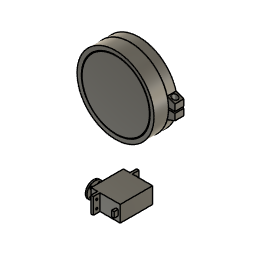
FlatPanel - SpaceCat51 v10 (Autodesk Fusion 360 design; units mm, degrees)
Autodesk Fusion 360 part; units mm, degrees
sketch "Sketch1" plane through (0, 0, 0) normal (0, 1, 0) x (1, 0, 0) in component "TelescopeBracket"
  circle A0 centre (0, 0) radius 40 construction
  circle A1 centre (0, 0) radius 42.4
  circle A2 centre (0, 0) radius 47.4
  line L0 (0, 0) -> (47.4, 0) construction
  line L1 (42.3882, -1) -> (48.4, -1)
  line L2 (48.4, -1) -> (48.4, 1)
  line L3 (48.4, 1) -> (42.3882, 1)
  line L4 (42.3882, 1) -> (42.3882, -1)
  line L5 (42.3882, -1) -> (55.3882, -1)
  line L6 (55.3882, -1) -> (55.3882, -4)
  line L7 (55.3882, -4) -> (42.3882, -4)
  line L8 (42.3882, -4) -> (42.3882, -1)
  line L9 (55.3882, -4) -> (42.3882, -4)
  line L10 (42.3882, -4) -> (42.3882, -9)
  line L11 (42.3882, -9) -> (55.3882, -9)
  line L12 (55.3882, -9) -> (55.3882, -4)
  line L13 (55.3882, -9) -> (45.7166, -12.5202)
  line L14 (55.3882, -9) -> (65.3491, -9) construction
  line L15 (42.3882, 1) -> (55.3882, 1)
  line L16 (55.3882, 1) -> (55.3882, 4)
  line L17 (55.3882, 9) -> (55.3882, 4)
  line L18 (55.3882, 9) -> (45.7166, 12.5202)
  dimension "d1" = 80
  dimension "d3" = 2.4
  dimension "d4" = 5
  dimension "d15" = 2
  dimension "d16" = 1
  dimension "d17" = 13
  dimension "d18" = 3
  dimension "d20" = 5
  dimension "d21" = 160
  constraint coincident A0.centre A1.centre
  constraint coincident A2 L0.end
  constraint horizontal L0
  constraint horizontal L1
  constraint vertical L2
  constraint horizontal L3
  constraint vertical L4
  constraint coincident A1 L1.start
  constraint horizontal L5
  constraint vertical L6
  constraint horizontal L7
  constraint vertical L8
  constraint horizontal L9
  constraint vertical L10
  constraint horizontal L11
  constraint vertical L12
  constraint horizontal L14
  constraint symmetric L0 L1.start L3.end
  constraint symmetric L0 L5.end L15.end
  constraint symmetric L0 L6.end L16.end
  constraint symmetric L0 L11.end L17.start
  constraint symmetric L0 L13.end L18.end
  constraint coincident A2 L13.end
  measures "d1" diameter of A0
  measures "d3" distance of A0 A1
  measures "d4" distance of A1 A2
  measures "d15" distance of L1 L3
  measures "d16" distance of L0 L1
  measures "d17" distance of L1.start L5.end
  measures "d18" distance of L5 L7
  measures "d20" distance of L6.end L11.end
  measures "d21" angle of L13 L14
extrude "Extrude2" add sketch "Sketch1" along normal blind 11 contours A1 A2 L3 L8 L10 L11 L15 | A2 L1 L5 L7 L8 L9 | A2 L3 L15 L16 L17 L18 | A2 L1 L5 L6 L7 L9 | A2 L7 L9 L10 L11 | A2 L7 L9 L11 L12 | A2 L11 L13 makes body 1 in component "TelescopeBracket"
sketch "Sketch2" plane through (0, 0, -1) normal (0, 0, 1) x (-1, 0, 0) in component "TelescopeBracket"
  line L0 (-42.3882, 0) -> (-55.3882, 0)
  line L1 (-55.3882, -11) -> (-42.3882, -11)
  line L2 (-42.3882, -11) -> (-42.3882, 0)
  circle A0 centre (-49.3882, -5.5) radius 3
  circle A1 centre (-49.3882, -5.5) radius 3
  line L3 (-55.3882, 0) -> (-55.3882, -11)
  dimension "d24" = 6
  dimension "d25" = 6
  dimension "d38" = 6
  dimension "d39" = 6
  dimension "d40" = 5.5
  dimension "d41" = 5.5
  measures "d24" diameter of A0
  measures "d25" diameter of A1
  measures "d38" distance of A0.centre L3
  measures "d39" distance of A0.centre L3
  measures "d40" distance of L0 A0.centre
  measures "d41" distance of L1 A0.centre
extrude "Extrude3" cut sketch "Sketch2" against normal blind 20 contours A0 A1 bodies 1 in component "TelescopeBracket"
sketch "Sketch3" plane through (0, 0, 1) normal (0, 0, -1) x (1, 0, 0) in component "TelescopeBracket"
  line L0 (55.3882, 0) -> (42.3882, 0)
  line L1 (42.3882, 0) -> (42.3882, -11)
  line L2 (42.3882, -11) -> (55.3882, -11)
  line L3 (55.3882, -11) -> (55.3882, 0)
  circle A0 centre (49.8882, -5.5) radius 2
  circle A1 centre (49.8882, -5.5) radius 2
  circle A2 centre (49.8882, -5.5) radius 3.5
  circle A3 centre (49.8882, -5.5) radius 3.5
  dimension "d30" = 4
  dimension "d31" = 4
  dimension "d32" = 7
  dimension "d33" = 7
  dimension "d44" = 5.5
  dimension "d45" = 5.5
  dimension "d46" = 5.5
  dimension "d47" = 5.5
  constraint concentric A0 A2
  constraint concentric A1 A3
  measures "d30" diameter of A0
  measures "d31" diameter of A1
  measures "d32" diameter of A2
  measures "d33" diameter of A3
  measures "d44" distance of L0 A0.centre
  measures "d45" distance of L2 A0.centre
  measures "d46" distance of L3 A0.centre
  measures "d47" distance of L3 A0.centre
extrude "Extrude4" cut sketch "Sketch3" against normal blind 20 contours A0 A1 | A2 A3 bodies 1 in component "TelescopeBracket"
extrude "Extrude5" add sketch "Sketch3" against normal blind 3 contours A2 A3 bodies 1 in component "TelescopeBracket"
sketch "Sketch1 (2)" plane through (0, 0, 0) normal (0, 0, 1) x (1, 0, 0) in component "ServoMockup"
  line L0 (0, 0) -> (20, 0)
  line L1 (20, 0) -> (20, 56.4)
  line L2 (20, 56.4) -> (0, 56.4)
  line L3 (0, 56.4) -> (0, 0)
  line L4 (20, 8.2) -> (0, 8.2)
  line L5 (0, 8.2) -> (0, 48.2)
  line L6 (0, 48.2) -> (20, 48.2)
  line L7 (20, 48.2) -> (20, 8.2)
  line L8 (20, 8.2) -> (0, 48.2) construction
  line L9 (0, 8.2) -> (20, 48.2) construction
  line L10 (15, 4.2) -> (5, 4.2) construction
  line L11 (5, 4.2) -> (5, 52.2) construction
  line L12 (5, 52.2) -> (15, 52.2) construction
  line L13 (15, 52.2) -> (15, 4.2) construction
  line L14 (15, 4.2) -> (5, 52.2) construction
  line L15 (5, 4.2) -> (15, 52.2) construction
  circle A0 centre (5, 52.2) radius 1.25
  circle A1 centre (15, 52.2) radius 1.25
  circle A2 centre (5, 4.2) radius 1.25
  circle A3 centre (15, 4.2) radius 1.25
  circle A4 centre (10, 38.2) radius 3
  point P0 (10, 28.2)
  point P1 (10, 28.2)
  dimension "d48" = 20
  dimension "d49" = 56.4
  dimension "d50" = 40
  dimension "d51" = 28.2
  dimension "d52" = 20
  dimension "d53" = 10
  dimension "d54" = 48
  dimension "d55" = 2.5
  dimension "d56" = 2.5
  dimension "d57" = 2.5
  dimension "d58" = 2.5
  dimension "d59" = 10
  dimension "d66" = 6
  dimension "d67" = 10
  dimension "d68" = 10
  constraint horizontal L0
  constraint vertical L1
  constraint horizontal L2
  constraint vertical L3
  constraint coincident L0.start L3.end
  constraint horizontal L4
  constraint perpendicular L4 L5
  constraint parallel L4 L6
  constraint parallel L5 L7
  constraint coincident L8 P1
  constraint coincident L9 P1
  constraint horizontal L10
  constraint perpendicular L10 L11
  constraint parallel L10 L12
  constraint parallel L11 L13
  constraint coincident L14 P1
  constraint coincident L15 P1
  constraint coincident P1 P0
  constraint coincident L11.end L12.start
  constraint coincident L12.end L13.start
  constraint coincident L10.end L11.start
  constraint coincident L10.start L13.end
  measures "d48" distance of L0.start L0.end
  measures "d49" distance of L0.start L2.end
  measures "d50" distance of L4.end L5.end
  measures "d51" distance of L2 P1
  measures "d52" distance of L1 L5
  measures "d53" distance of L11.end L12.end
  measures "d54" distance of L10.end L11.end
  measures "d55" diameter of A0
  measures "d56" diameter of A1
  measures "d57" diameter of A2
  measures "d58" diameter of A3
  measures "d59" distance of L3 P1
  measures "d66" diameter of A4
  measures "d67" distance of L3 A4.centre
  measures "d68" distance of L6 A4.centre
extrude "Extrude1" add sketch "Sketch1 (2)" against normal blind 25 separate body contours L1 L3 L4 L5 L6 L7 | A4 makes body 2 in component "ServoMockup"
extrude "Extrude2'" add sketch "Sketch1 (2)" along normal blind 3 contours L0 L1 L3 L4 | L1 L3 L4 L5 L6 L7 | L1 L2 L3 L6 | A4 bodies 2 in component "ServoMockup"
extrude "Extrude3'" add sketch "Sketch1 (2)" along normal blind 11 contours L1 L3 L4 L5 L6 L7 | A4 bodies 2 in component "ServoMockup"
extrude "Extrude4'" add sketch "Sketch1 (2)" along normal blind 16 contours A4 bodies 2 in component "ServoMockup"
sketch "Sketch2 (2)" plane through (0, 0, 16) normal (0, 0, 1) x (-1, 0, 0) in component "ServoMockup"
  circle A0 centre (-10, -38.2) radius 3
  circle A1 centre (-10, -38.2) radius 10
  line L0 (-15, -43.2) -> (-5, -43.2) construction
  line L1 (-5, -43.2) -> (-5, -33.2) construction
  line L2 (-5, -33.2) -> (-15, -33.2) construction
  line L3 (-15, -33.2) -> (-15, -43.2) construction
  line L4 (-15, -43.2) -> (-5, -33.2) construction
  line L5 (-5, -43.2) -> (-15, -33.2) construction
  circle A2 centre (-5, -33.2) radius 1.5
  circle A3 centre (-5, -43.2) radius 1.5
  circle A4 centre (-15, -43.2) radius 1.5
  circle A5 centre (-15, -33.2) radius 1.5
  circle A6 centre (-10, -38.2) radius 4.75
  circle A7 centre (-10, -38.2) radius 1.5
  point P0 (-10, -38.2)
  dimension "d71" = 20
  dimension "d72" = 10
  dimension "d73" = 10
  dimension "d74" = 3
  dimension "d75" = 3
  dimension "d76" = 3
  dimension "d77" = 3
  dimension "d78" = 9.5
  dimension "d81" = 3
  constraint concentric A0 A1
  constraint horizontal L0
  constraint perpendicular L0 L1
  constraint parallel L0 L2
  constraint parallel L1 L3
  constraint coincident L4 P0
  constraint coincident L5 P0
  constraint coincident P0 A0.centre
  constraint coincident L1.end L2.start
  constraint coincident L0.end L1.start
  constraint coincident L0.start L3.end
  constraint coincident L2.end L3.start
  constraint concentric A1 A6
  constraint concentric A6 A7
  measures "d71" diameter of A1
  measures "d72" distance of L1.end L2.end
  measures "d73" distance of L0.end L1.end
  measures "d74" diameter of A2
  measures "d75" diameter of A3
  measures "d76" diameter of A4
  measures "d77" diameter of A5
  measures "d78" diameter of A6
  measures "d81" diameter of A7
extrude "Extrude5'" add sketch "Sketch2 (2)" against normal blind 3 separate body contours A6 makes body 3 in component "ServoMockup"
extrude "Extrude6" add sketch "Sketch2 (2)" along normal blind 2 contours A0 | A1 | A6 bodies 3 in component "ServoMockup"
sketch "Sketch3 (2)" plane through (0, 48.2, 0) normal (0, 1, 0) x (-1, 0, 0) in component "ServoMockup"
  line L0 (0, 0) -> (-20, 0)
  line L1 (-20, 0) -> (-20, -25)
  line L2 (-20, -25) -> (0, -25)
  line L3 (0, -25) -> (0, 0)
  line L4 (-13.5, -19.5) -> (-6.5, -19.5)
  line L5 (-6.5, -19.5) -> (-6.5, -22.5)
  line L6 (-6.5, -22.5) -> (-13.5, -22.5)
  line L7 (-13.5, -22.5) -> (-13.5, -19.5)
  dimension "d84" = 7
  dimension "d85" = 3
  dimension "d86" = 2.5
  dimension "d87" = 6.5
  constraint horizontal L4
  constraint vertical L5
  constraint horizontal L6
  constraint vertical L7
  measures "d84" distance of L5 L7
  measures "d85" distance of L4 L6
  measures "d86" distance of L2 L6
  measures "d87" distance of L1 L7
extrude "Extrude7" add sketch "Sketch3 (2)" along normal blind 5 contours L4 L5 L6 L7 bodies 2 in component "ServoMockup"
sketch "Sketch1 (3)" plane through (0, 0, 0) normal (0, 1, 0) x (1, 0, 0) in component "FlatPanelHousing"
  circle A0 centre (0, 0) radius 40
  circle A1 centre (0, 0) radius 42.5
  circle A2 centre (0, 0) radius 47.5
  circle A3 centre (0, 0) radius 44.5
  dimension "d90" = 80
  dimension "d91" = 85
  dimension "d92" = 95
  dimension "d99" = 89
  constraint coincident A0.centre A1.centre
  constraint concentric A1 A2
  constraint concentric A1 A3
  measures "d90" diameter of A0
  measures "d91" diameter of A1
  measures "d92" diameter of A2
  measures "d99" diameter of A3
extrude "Extrude1'" add sketch "Sketch1 (3)" against normal blind 18 separate body contours A0 | A1 | A2 | A3 makes body 4 in component "FlatPanelHousing"
extrude "Extrude4''" cut sketch "Sketch1 (3)" against normal blind 15 contours A0 | A1 bodies 4 in component "FlatPanelHousing"
extrude "Extrude5''" cut sketch "Sketch1 (3)" against normal blind 12 contours A3 bodies 4 in component "FlatPanelHousing"
extrude "Extrude6'" add sketch "Sketch1 (3)" against normal blind 7 contours A3 bodies 4 in component "FlatPanelHousing"
extrude "Extrude7'" add sketch "Sketch1 (3)" against normal blind 3 contours A1 bodies 4 in component "FlatPanelHousing"
extrude "Extrude8" add sketch "Sketch1 (3)" against normal blind 3 separate body contours A0 | A1 makes body 5 in component "FlatPanelHousing"
move_body "Move1" bodies 5 to x (1, 0, 0) y (0, 1, 0) z (0, 0, 1) at (0, -12, 0) in component "FlatPanelHousing"
extrude "Extrude9" add sketch "Sketch1 (3)" against normal blind 5 separate body contours A0 | A1 makes body 6 in component "FlatPanelHousing"
move_body "Move2" bodies 6 to x (1, 0, 0) y (0, 1, 0) z (0, 0, 1) at (0, -7, 0) in component "FlatPanelHousing"
extrude "Extrude10" add sketch "Sketch1 (3)" against normal blind 3 separate body contours A0 | A1 makes body 7 in component "FlatPanelHousing"
move_body "Move3" bodies 7 to x (1, 0, 0) y (0, 1, 0) z (0, 0, 1) at (0, -4, 0) in component "FlatPanelHousing"
extrude "Extrude11" cut 1 faces at (8.8328, -15, 6.8531) along direction (0, -1, 0) up to surface (3 mm away) on bodies 4 bodies 4 in component "FlatPanelHousing"
extrude "Extrude12" add 1 faces at (8.8328, -15, 6.8531) along direction (0, -1, 0) blind 3 separate body on bodies 5 makes body 8 in component "FlatPanelHousing"
thread "Thread2" "ISO Metric profile 85.0 M85x1.5 6g" major diameter 84.85 minor diameter 83.1269 pitch 1.5 angle 60 modelled right hand crest width 0.2094 on face at (42.4472, -17, 2.1185) crest through (42.425, -14.625, 0) on bodies 8 in component "FlatPanelHousing"
thread "Thread3" "ISO Metric profile 85.0 M85x1.5 6H" major diameter 85.2143 minor diameter 83.5262 pitch 1.5 angle 60 modelled right hand crest width 0.4004 on face at (42.4472, -16, 2.1185) crest through (41.7631, -12.375, 0) on bodies 4 in component "FlatPanelHousing"
component "TelescopeBracket" placed x (1, 0, 0) y (0, 1, 0) z (0, 0, 1) at (0, 0, 0)
component "ServoMockup" placed x (0, 0, -1) y (0, -1, 0) z (-1, 0, 0) at (-10.6879, 21.6762, -105.6879)
component "FlatPanelHousing" placed x (1, 0, 0) y (0, 1, 0) z (0, 0, 1) at (0, 0, 0)
equation "d1 = TelescopeDiameter"
equation "TelescopeDiameter = 80 mm" comment "This is the diameter of the outside case of the telescopes main apeture where the ring will clamp against, providing the main connection"
equation "MagnetWidth = 6 mm" comment "Width of the front face of the circular magnets"
equation "d16 = d15 / 2"
equation "d17 = d4 + 8 mm"
equation "d38 = ( d25 / 2 ) + 3 mm"
equation "d39 = d38"
equation "d40 = ( 22 / 4 ) * 1 mm"
equation "d41 = d40"
equation "d44 = d40"
equation "d45 = d40"
equation "d46 = d40"
equation "d47 = d40"
equation "d51 = d49 / 2"
equation "d56 = d55"
equation "d57 = d55"
equation "d58 = d55"
equation "d62 = 3 mm"
equation "d64 = d62 + 8 mm"
equation "d69 = d64 + 5 mm"
equation "d87 = 10 mm - d84 / 2"
equation "d90 = TelescopeDiameter"
equation "d91 = d90 + 5 mm"
equation "d92 = d90 + 15 mm"
equation "d99 = d90 + 9 mm"
equation "d104 = -12 mm + 5 mm"
named bodies: "Servo", "ServoArm", "FlatPanelHousing", "MirrorPanel", "5mm Frosted Perspex", "3mm Frosted Perspex", "FlatPanelCap"
